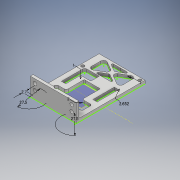
# Autodesk Inventor part: OpenMV&Ping
Saved by Autodesk Inventor 2018 (Build 220112000, 112)
## iProperties
Created: 2018-10-24
Part Number: OpenMV&Ping
Material: 一般
Document SubType Name: Modeling
Designer: shun2
Density: 1 g/cm^3
Appearance: 既定
Author: shun2
Autodesk Inventor part; units mm, degrees
ref_plane "YZ Plane" through (0, 0, 0) normal (1, 0, 0) x (0, 1, 0)
ref_plane "XZ Plane" through (0, 0, 0) normal (0, 1, 0) x (-1, 0, 0)
ref_plane "XY Plane" through (0, 0, 0) normal (0, 0, 1) x (1, 0, 0)
ref_plane "作業平面3" through (0, 0, 0) normal (0, 0, -1) x (-1, 0, 0)
sketch "スケッチ17" plane through (0, 0, 0) normal (0, 0, -1) x (-1, 0, 0)
  line L0 (19.0039, 20.5342) -> (19.0039, -23.9158)
  line L1 (19.0979, -0.4088) -> (19.0979, -12.4088)
  arc A0 (19.0661, -12.4088) -> (19.1297, -12.4088) centre (19.0979, -12.4088) ccw
  arc A1 (19.1297, -0.4088) -> (19.0661, -0.4088) centre (19.0979, -0.4088) ccw
  arc A2 (19.0979, -12.3771) -> (19.0979, -12.4406) centre (19.0979, -12.4088) ccw
  arc A3 (19.0979, -0.3771) -> (19.0979, -0.4406) centre (19.0979, -0.4088) ccw
  line L2 (1.4119, 34.5042) -> (1.4119, 35.1392)
  line L3 (-16.3681, -23.9158) -> (-16.3681, 20.5342)
  line L4 (-16.3681, 20.5342) -> (19.0039, 20.5342)
  line L5 (19.0039, -23.9158) -> (-16.3681, -23.9158)
  arc A4 (-15.9871, -20.6011) -> (-15.9871, -20.6265) centre (-15.9871, -20.6138) ccw
  arc A5 (-10.1451, -20.6265) -> (-10.1451, -20.6011) centre (-10.1451, -20.6138) ccw
  arc A6 (-13.0661, -23.5348) -> (-13.0661, -17.6928) centre (-13.0661, -20.6138) ccw
  arc A7 (-13.0661, -17.6928) -> (-13.0661, -23.5348) centre (-13.0661, -20.6138) ccw
  arc A8 (-13.0661, -22.1138) -> (-13.0661, -19.1138) centre (-13.0661, -20.6138) ccw
  arc A9 (-13.0661, -19.1138) -> (-13.0661, -22.1138) centre (-13.0661, -20.6138) ccw
  line L6 (18.8109, -20.6138) -> (18.5569, -20.6138)
  arc A10 (18.5569, -20.6011) -> (18.5569, -20.6265) centre (18.5569, -20.6138) ccw
  arc A11 (18.8109, -20.6265) -> (18.8109, -20.6011) centre (18.8109, -20.6138) ccw
  arc A12 (12.9689, -20.6011) -> (12.9689, -20.6265) centre (12.9689, -20.6138) ccw
  arc A13 (15.8899, -23.5348) -> (15.8899, -17.6928) centre (15.8899, -20.6138) ccw
  arc A14 (15.8899, -17.6928) -> (15.8899, -23.5348) centre (15.8899, -20.6138) ccw
  arc A15 (15.8899, -22.1138) -> (15.8899, -19.1138) centre (15.8899, -20.6138) ccw
  arc A16 (15.8899, -19.1138) -> (15.8899, -22.1138) centre (15.8899, -20.6138) ccw
  line L7 (18.8109, 15.8352) -> (18.8109, 17.1052)
  arc A17 (18.849, 17.1052) -> (18.7728, 17.1052) centre (18.8109, 17.1052) ccw
  arc A18 (18.7728, 15.8352) -> (18.849, 15.8352) centre (18.8109, 15.8352) ccw
  line L8 (18.8109, 17.1052) -> (18.1759, 17.7402)
  arc A19 (18.2028, 17.7671) -> (18.149, 17.7133) centre (18.1759, 17.7402) ccw
  arc A20 (18.784, 17.0783) -> (18.8378, 17.1321) centre (18.8109, 17.1052) ccw
  arc A21 (16.9059, 17.7783) -> (16.9059, 17.7021) centre (16.9059, 17.7402) ccw
  arc A22 (18.1759, 17.7021) -> (18.1759, 17.7783) centre (18.1759, 17.7402) ccw
  line L9 (16.9059, 17.7402) -> (16.2709, 17.1052)
  arc A23 (16.244, 17.1321) -> (16.2978, 17.0783) centre (16.2709, 17.1052) ccw
  arc A24 (16.9328, 17.7133) -> (16.879, 17.7671) centre (16.9059, 17.7402) ccw
  line L10 (18.1759, 12.6602) -> (18.8109, 13.2952)
  arc A25 (18.8378, 13.2683) -> (18.784, 13.3221) centre (18.8109, 13.2952) ccw
  arc A26 (18.149, 12.6871) -> (18.2028, 12.6333) centre (18.1759, 12.6602) ccw
  line L11 (18.8109, 13.2952) -> (18.8109, 14.5652)
  arc A27 (18.849, 14.5652) -> (18.7728, 14.5652) centre (18.8109, 14.5652) ccw
  arc A28 (18.7728, 13.2952) -> (18.849, 13.2952) centre (18.8109, 13.2952) ccw
  line L12 (18.8109, 14.5652) -> (18.1759, 15.2002)
  arc A29 (18.2028, 15.2271) -> (18.149, 15.1733) centre (18.1759, 15.2002) ccw
  arc A30 (18.784, 14.5383) -> (18.8378, 14.5921) centre (18.8109, 14.5652) ccw
  arc A31 (16.9059, 15.2383) -> (16.9059, 15.1621) centre (16.9059, 15.2002) ccw
  arc A32 (18.1759, 15.1621) -> (18.1759, 15.2383) centre (18.1759, 15.2002) ccw
  line L13 (16.9059, 15.2002) -> (16.2709, 14.5652)
  arc A33 (16.244, 14.5921) -> (16.2978, 14.5383) centre (16.2709, 14.5652) ccw
  arc A34 (16.9328, 15.1733) -> (16.879, 15.2271) centre (16.9059, 15.2002) ccw
  line L14 (16.2709, 14.5652) -> (16.2709, 13.2952)
  arc A35 (16.2328, 13.2952) -> (16.309, 13.2952) centre (16.2709, 13.2952) ccw
  arc A36 (16.309, 14.5652) -> (16.2328, 14.5652) centre (16.2709, 14.5652) ccw
  line L15 (16.2709, 13.2952) -> (16.9059, 12.6602)
  arc A37 (16.879, 12.6333) -> (16.9328, 12.6871) centre (16.9059, 12.6602) ccw
  arc A38 (16.2978, 13.3221) -> (16.244, 13.2683) centre (16.2709, 13.2952) ccw
  line L16 (18.8109, 15.8352) -> (18.1759, 15.2002)
  arc A39 (18.149, 15.2271) -> (18.2028, 15.1733) centre (18.1759, 15.2002) ccw
  arc A40 (18.8378, 15.8083) -> (18.784, 15.8621) centre (18.8109, 15.8352) ccw
  line L17 (16.9059, 15.2002) -> (16.2709, 15.8352)
  arc A41 (16.2978, 15.8621) -> (16.244, 15.8083) centre (16.2709, 15.8352) ccw
  arc A42 (16.879, 15.1733) -> (16.9328, 15.2271) centre (16.9059, 15.2002) ccw
  line L18 (16.2709, 17.1052) -> (16.2709, 15.8352)
  arc A43 (16.2328, 15.8352) -> (16.309, 15.8352) centre (16.2709, 15.8352) ccw
  arc A44 (16.309, 17.1052) -> (16.2328, 17.1052) centre (16.2709, 17.1052) ccw
  line L19 (18.8109, 8.2152) -> (18.8109, 9.4852)
  arc A45 (18.849, 9.4852) -> (18.7728, 9.4852) centre (18.8109, 9.4852) ccw
  arc A46 (18.7728, 8.2152) -> (18.849, 8.2152) centre (18.8109, 8.2152) ccw
  line L20 (18.8109, 9.4852) -> (18.1759, 10.1202)
  arc A47 (18.2028, 10.1471) -> (18.149, 10.0933) centre (18.1759, 10.1202) ccw
  arc A48 (18.784, 9.4583) -> (18.8378, 9.5121) centre (18.8109, 9.4852) ccw
  arc A49 (16.9059, 10.1583) -> (16.9059, 10.0821) centre (16.9059, 10.1202) ccw
  arc A50 (18.1759, 10.0821) -> (18.1759, 10.1583) centre (18.1759, 10.1202) ccw
  line L21 (16.9059, 10.1202) -> (16.2709, 9.4852)
  arc A51 (16.244, 9.5121) -> (16.2978, 9.4583) centre (16.2709, 9.4852) ccw
  arc A52 (16.9328, 10.0933) -> (16.879, 10.1471) centre (16.9059, 10.1202) ccw
  line L22 (18.1759, 10.1202) -> (18.8109, 10.7552)
  arc A53 (18.8378, 10.7283) -> (18.784, 10.7821) centre (18.8109, 10.7552) ccw
  arc A54 (18.149, 10.1471) -> (18.2028, 10.0933) centre (18.1759, 10.1202) ccw
  line L23 (18.8109, 10.7552) -> (18.8109, 12.0252)
  arc A55 (18.849, 12.0252) -> (18.7728, 12.0252) centre (18.8109, 12.0252) ccw
  arc A56 (18.7728, 10.7552) -> (18.849, 10.7552) centre (18.8109, 10.7552) ccw
  line L24 (18.8109, 12.0252) -> (18.1759, 12.6602)
  arc A57 (18.2028, 12.6871) -> (18.149, 12.6333) centre (18.1759, 12.6602) ccw
  arc A58 (18.784, 11.9983) -> (18.8378, 12.0521) centre (18.8109, 12.0252) ccw
  arc A59 (16.9059, 12.6983) -> (16.9059, 12.6221) centre (16.9059, 12.6602) ccw
  arc A60 (18.1759, 12.6221) -> (18.1759, 12.6983) centre (18.1759, 12.6602) ccw
  line L25 (16.9059, 12.6602) -> (16.2709, 12.0252)
  arc A61 (16.244, 12.0521) -> (16.2978, 11.9983) centre (16.2709, 12.0252) ccw
  arc A62 (16.9328, 12.6333) -> (16.879, 12.6871) centre (16.9059, 12.6602) ccw
  line L26 (16.2709, 12.0252) -> (16.2709, 10.7552)
  arc A63 (16.2328, 10.7552) -> (16.309, 10.7552) centre (16.2709, 10.7552) ccw
  arc A64 (16.309, 12.0252) -> (16.2328, 12.0252) centre (16.2709, 12.0252) ccw
  line L27 (16.2709, 10.7552) -> (16.9059, 10.1202)
  arc A65 (16.879, 10.0933) -> (16.9328, 10.1471) centre (16.9059, 10.1202) ccw
  arc A66 (16.2978, 10.7821) -> (16.244, 10.7283) centre (16.2709, 10.7552) ccw
  line L28 (18.1759, 5.0402) -> (18.8109, 5.6752)
  arc A67 (18.8378, 5.6483) -> (18.784, 5.7021) centre (18.8109, 5.6752) ccw
  arc A68 (18.149, 5.0671) -> (18.2028, 5.0133) centre (18.1759, 5.0402) ccw
  line L29 (18.8109, 5.6752) -> (18.8109, 6.9452)
  arc A69 (18.849, 6.9452) -> (18.7728, 6.9452) centre (18.8109, 6.9452) ccw
  arc A70 (18.7728, 5.6752) -> (18.849, 5.6752) centre (18.8109, 5.6752) ccw
  line L30 (18.8109, 6.9452) -> (18.1759, 7.5802)
  arc A71 (18.2028, 7.6071) -> (18.149, 7.5533) centre (18.1759, 7.5802) ccw
  arc A72 (18.784, 6.9183) -> (18.8378, 6.9721) centre (18.8109, 6.9452) ccw
  arc A73 (16.9059, 7.6183) -> (16.9059, 7.5421) centre (16.9059, 7.5802) ccw
  arc A74 (18.1759, 7.5421) -> (18.1759, 7.6183) centre (18.1759, 7.5802) ccw
  line L31 (16.9059, 7.5802) -> (16.2709, 6.9452)
  arc A75 (16.244, 6.9721) -> (16.2978, 6.9183) centre (16.2709, 6.9452) ccw
  arc A76 (16.9328, 7.5533) -> (16.879, 7.6071) centre (16.9059, 7.5802) ccw
  line L32 (16.2709, 6.9452) -> (16.2709, 5.6752)
  arc A77 (16.2328, 5.6752) -> (16.309, 5.6752) centre (16.2709, 5.6752) ccw
  arc A78 (16.309, 6.9452) -> (16.2328, 6.9452) centre (16.2709, 6.9452) ccw
  line L33 (16.2709, 5.6752) -> (16.9059, 5.0402)
  arc A79 (16.879, 5.0133) -> (16.9328, 5.0671) centre (16.9059, 5.0402) ccw
  arc A80 (16.2978, 5.7021) -> (16.244, 5.6483) centre (16.2709, 5.6752) ccw
  line L34 (18.8109, 8.2152) -> (18.1759, 7.5802)
  arc A81 (18.149, 7.6071) -> (18.2028, 7.5533) centre (18.1759, 7.5802) ccw
  arc A82 (18.8378, 8.1883) -> (18.784, 8.2421) centre (18.8109, 8.2152) ccw
  line L35 (16.9059, 7.5802) -> (16.2709, 8.2152)
  arc A83 (16.2978, 8.2421) -> (16.244, 8.1883) centre (16.2709, 8.2152) ccw
  arc A84 (16.879, 7.5533) -> (16.9328, 7.6071) centre (16.9059, 7.5802) ccw
  line L36 (16.2709, 9.4852) -> (16.2709, 8.2152)
  arc A85 (16.2328, 8.2152) -> (16.309, 8.2152) centre (16.2709, 8.2152) ccw
  arc A86 (16.309, 9.4852) -> (16.2328, 9.4852) centre (16.2709, 9.4852) ccw
  line L37 (18.8109, 0.5952) -> (18.8109, 1.8652)
  arc A87 (18.849, 1.8652) -> (18.7728, 1.8652) centre (18.8109, 1.8652) ccw
  arc A88 (18.7728, 0.5952) -> (18.849, 0.5952) centre (18.8109, 0.5952) ccw
  line L38 (18.8109, 1.8652) -> (18.1759, 2.5002)
  arc A89 (18.2028, 2.5271) -> (18.149, 2.4733) centre (18.1759, 2.5002) ccw
  arc A90 (18.784, 1.8383) -> (18.8378, 1.8921) centre (18.8109, 1.8652) ccw
  arc A91 (16.9059, 2.5383) -> (16.9059, 2.4621) centre (16.9059, 2.5002) ccw
  arc A92 (18.1759, 2.4621) -> (18.1759, 2.5383) centre (18.1759, 2.5002) ccw
  line L39 (16.9059, 2.5002) -> (16.2709, 1.8652)
  arc A93 (16.244, 1.8921) -> (16.2978, 1.8383) centre (16.2709, 1.8652) ccw
  arc A94 (16.9328, 2.4733) -> (16.879, 2.5271) centre (16.9059, 2.5002) ccw
  line L40 (18.1759, 2.5002) -> (18.8109, 3.1352)
  arc A95 (18.8378, 3.1083) -> (18.784, 3.1621) centre (18.8109, 3.1352) ccw
  arc A96 (18.149, 2.5271) -> (18.2028, 2.4733) centre (18.1759, 2.5002) ccw
  line L41 (18.8109, 3.1352) -> (18.8109, 4.4052)
  arc A97 (18.849, 4.4052) -> (18.7728, 4.4052) centre (18.8109, 4.4052) ccw
  arc A98 (18.7728, 3.1352) -> (18.849, 3.1352) centre (18.8109, 3.1352) ccw
  line L42 (18.8109, 4.4052) -> (18.1759, 5.0402)
  arc A99 (18.2028, 5.0671) -> (18.149, 5.0133) centre (18.1759, 5.0402) ccw
  arc A100 (18.784, 4.3783) -> (18.8378, 4.4321) centre (18.8109, 4.4052) ccw
  arc A101 (16.9059, 5.0783) -> (16.9059, 5.0021) centre (16.9059, 5.0402) ccw
  arc A102 (18.1759, 5.0021) -> (18.1759, 5.0783) centre (18.1759, 5.0402) ccw
  line L43 (16.9059, 5.0402) -> (16.2709, 4.4052)
  arc A103 (16.244, 4.4321) -> (16.2978, 4.3783) centre (16.2709, 4.4052) ccw
  arc A104 (16.9328, 5.0133) -> (16.879, 5.0671) centre (16.9059, 5.0402) ccw
  line L44 (16.2709, 4.4052) -> (16.2709, 3.1352)
  arc A105 (16.2328, 3.1352) -> (16.309, 3.1352) centre (16.2709, 3.1352) ccw
  arc A106 (16.309, 4.4052) -> (16.2328, 4.4052) centre (16.2709, 4.4052) ccw
  line L45 (16.2709, 3.1352) -> (16.9059, 2.5002)
  arc A107 (16.879, 2.4733) -> (16.9328, 2.5271) centre (16.9059, 2.5002) ccw
  arc A108 (16.2978, 3.1621) -> (16.244, 3.1083) centre (16.2709, 3.1352) ccw
  line L46 (18.1759, -0.0398) -> (16.9059, -0.0398)
  arc A109 (16.9059, -0.0017) -> (16.9059, -0.0779) centre (16.9059, -0.0398) ccw
  arc A110 (18.1759, -0.0779) -> (18.1759, -0.0017) centre (18.1759, -0.0398) ccw
  line L47 (18.8109, 0.5952) -> (18.1759, -0.0398)
  arc A111 (18.149, -0.0129) -> (18.2028, -0.0667) centre (18.1759, -0.0398) ccw
  arc A112 (18.8378, 0.5683) -> (18.784, 0.6221) centre (18.8109, 0.5952) ccw
  line L48 (16.9059, -0.0398) -> (16.2709, 0.5952)
  arc A113 (16.2978, 0.6221) -> (16.244, 0.5683) centre (16.2709, 0.5952) ccw
  arc A114 (16.879, -0.0667) -> (16.9328, -0.0129) centre (16.9059, -0.0398) ccw
  line L49 (16.2709, 1.8652) -> (16.2709, 0.5952)
  arc A115 (16.2328, 0.5952) -> (16.309, 0.5952) centre (16.2709, 0.5952) ccw
  arc A116 (16.309, 1.8652) -> (16.2328, 1.8652) centre (16.2709, 1.8652) ccw
  line L50 (18.8109, 18.3752) -> (18.8109, 19.6452)
  arc A117 (18.849, 19.6452) -> (18.7728, 19.6452) centre (18.8109, 19.6452) ccw
  arc A118 (18.7728, 18.3752) -> (18.849, 18.3752) centre (18.8109, 18.3752) ccw
  line L51 (18.8109, 19.6452) -> (18.1759, 20.2802)
  arc A119 (18.2028, 20.3071) -> (18.149, 20.2533) centre (18.1759, 20.2802) ccw
  arc A120 (18.784, 19.6183) -> (18.8378, 19.6721) centre (18.8109, 19.6452) ccw
  line L52 (18.1759, 20.2802) -> (16.9059, 20.2802)
  arc A121 (16.9059, 20.3183) -> (16.9059, 20.2421) centre (16.9059, 20.2802) ccw
  arc A122 (18.1759, 20.2421) -> (18.1759, 20.3183) centre (18.1759, 20.2802) ccw
  line L53 (16.9059, 20.2802) -> (16.2709, 19.6452)
  arc A123 (16.244, 19.6721) -> (16.2978, 19.6183) centre (16.2709, 19.6452) ccw
  arc A124 (16.9328, 20.2533) -> (16.879, 20.3071) centre (16.9059, 20.2802) ccw
  line L54 (18.8109, 18.3752) -> (18.1759, 17.7402)
  arc A125 (18.149, 17.7671) -> (18.2028, 17.7133) centre (18.1759, 17.7402) ccw
  arc A126 (18.8378, 18.3483) -> (18.784, 18.4021) centre (18.8109, 18.3752) ccw
  line L55 (16.9059, 17.7402) -> (16.2709, 18.3752)
  arc A127 (16.2978, 18.4021) -> (16.244, 18.3483) centre (16.2709, 18.3752) ccw
  arc A128 (16.879, 17.7133) -> (16.9328, 17.7671) centre (16.9059, 17.7402) ccw
  line L56 (16.2709, 19.6452) -> (16.2709, 18.3752)
  arc A129 (16.2328, 18.3752) -> (16.309, 18.3752) centre (16.2709, 18.3752) ccw
  arc A130 (16.309, 19.6452) -> (16.2328, 19.6452) centre (16.2709, 19.6452) ccw
  line L57 (-13.4471, 15.8352) -> (-13.4471, 17.1052)
  arc A131 (-13.409, 17.1052) -> (-13.4852, 17.1052) centre (-13.4471, 17.1052) ccw
  arc A132 (-13.4852, 15.8352) -> (-13.409, 15.8352) centre (-13.4471, 15.8352) ccw
  line L58 (-13.4471, 17.1052) -> (-14.0821, 17.7402)
  arc A133 (-14.0552, 17.7671) -> (-14.109, 17.7133) centre (-14.0821, 17.7402) ccw
  arc A134 (-13.474, 17.0783) -> (-13.4202, 17.1321) centre (-13.4471, 17.1052) ccw
  arc A135 (-15.3521, 17.7783) -> (-15.3521, 17.7021) centre (-15.3521, 17.7402) ccw
  arc A136 (-14.0821, 17.7021) -> (-14.0821, 17.7783) centre (-14.0821, 17.7402) ccw
  line L59 (-15.3521, 17.7402) -> (-15.9871, 17.1052)
  arc A137 (-16.014, 17.1321) -> (-15.9602, 17.0783) centre (-15.9871, 17.1052) ccw
  arc A138 (-15.3252, 17.7133) -> (-15.379, 17.7671) centre (-15.3521, 17.7402) ccw
  line L60 (-14.0821, 12.6602) -> (-13.4471, 13.2952)
  arc A139 (-13.4202, 13.2683) -> (-13.474, 13.3221) centre (-13.4471, 13.2952) ccw
  arc A140 (-14.109, 12.6871) -> (-14.0552, 12.6333) centre (-14.0821, 12.6602) ccw
  line L61 (-13.4471, 13.2952) -> (-13.4471, 14.5652)
  arc A141 (-13.409, 14.5652) -> (-13.4852, 14.5652) centre (-13.4471, 14.5652) ccw
  arc A142 (-13.4852, 13.2952) -> (-13.409, 13.2952) centre (-13.4471, 13.2952) ccw
  line L62 (-13.4471, 14.5652) -> (-14.0821, 15.2002)
  arc A143 (-14.0552, 15.2271) -> (-14.109, 15.1733) centre (-14.0821, 15.2002) ccw
  arc A144 (-13.474, 14.5383) -> (-13.4202, 14.5921) centre (-13.4471, 14.5652) ccw
  arc A145 (-15.3521, 15.2383) -> (-15.3521, 15.1621) centre (-15.3521, 15.2002) ccw
  arc A146 (-14.0821, 15.1621) -> (-14.0821, 15.2383) centre (-14.0821, 15.2002) ccw
  line L63 (-15.3521, 15.2002) -> (-15.9871, 14.5652)
  arc A147 (-16.014, 14.5921) -> (-15.9602, 14.5383) centre (-15.9871, 14.5652) ccw
  arc A148 (-15.3252, 15.1733) -> (-15.379, 15.2271) centre (-15.3521, 15.2002) ccw
  line L64 (-15.9871, 14.5652) -> (-15.9871, 13.2952)
  arc A149 (-16.0252, 13.2952) -> (-15.949, 13.2952) centre (-15.9871, 13.2952) ccw
  arc A150 (-15.949, 14.5652) -> (-16.0252, 14.5652) centre (-15.9871, 14.5652) ccw
  line L65 (-15.9871, 13.2952) -> (-15.3521, 12.6602)
  arc A151 (-15.379, 12.6333) -> (-15.3252, 12.6871) centre (-15.3521, 12.6602) ccw
  arc A152 (-15.9602, 13.3221) -> (-16.014, 13.2683) centre (-15.9871, 13.2952) ccw
  line L66 (-13.4471, 15.8352) -> (-14.0821, 15.2002)
  arc A153 (-14.109, 15.2271) -> (-14.0552, 15.1733) centre (-14.0821, 15.2002) ccw
  arc A154 (-13.4202, 15.8083) -> (-13.474, 15.8621) centre (-13.4471, 15.8352) ccw
  line L67 (-15.3521, 15.2002) -> (-15.9871, 15.8352)
  arc A155 (-15.9602, 15.8621) -> (-16.014, 15.8083) centre (-15.9871, 15.8352) ccw
  arc A156 (-15.379, 15.1733) -> (-15.3252, 15.2271) centre (-15.3521, 15.2002) ccw
  line L68 (-15.9871, 17.1052) -> (-15.9871, 15.8352)
  arc A157 (-16.0252, 15.8352) -> (-15.949, 15.8352) centre (-15.9871, 15.8352) ccw
  arc A158 (-15.949, 17.1052) -> (-16.0252, 17.1052) centre (-15.9871, 17.1052) ccw
  line L69 (-13.4471, 8.2152) -> (-13.4471, 9.4852)
  arc A159 (-13.409, 9.4852) -> (-13.4852, 9.4852) centre (-13.4471, 9.4852) ccw
  arc A160 (-13.4852, 8.2152) -> (-13.409, 8.2152) centre (-13.4471, 8.2152) ccw
  line L70 (-13.4471, 9.4852) -> (-14.0821, 10.1202)
  arc A161 (-14.0552, 10.1471) -> (-14.109, 10.0933) centre (-14.0821, 10.1202) ccw
  arc A162 (-13.474, 9.4583) -> (-13.4202, 9.5121) centre (-13.4471, 9.4852) ccw
  arc A163 (-15.3521, 10.1583) -> (-15.3521, 10.0821) centre (-15.3521, 10.1202) ccw
  arc A164 (-14.0821, 10.0821) -> (-14.0821, 10.1583) centre (-14.0821, 10.1202) ccw
  line L71 (-15.3521, 10.1202) -> (-15.9871, 9.4852)
  arc A165 (-16.014, 9.5121) -> (-15.9602, 9.4583) centre (-15.9871, 9.4852) ccw
  arc A166 (-15.3252, 10.0933) -> (-15.379, 10.1471) centre (-15.3521, 10.1202) ccw
  line L72 (-14.0821, 10.1202) -> (-13.4471, 10.7552)
  arc A167 (-13.4202, 10.7283) -> (-13.474, 10.7821) centre (-13.4471, 10.7552) ccw
  arc A168 (-14.109, 10.1471) -> (-14.0552, 10.0933) centre (-14.0821, 10.1202) ccw
  line L73 (-13.4471, 10.7552) -> (-13.4471, 12.0252)
  arc A169 (-13.409, 12.0252) -> (-13.4852, 12.0252) centre (-13.4471, 12.0252) ccw
  arc A170 (-13.4852, 10.7552) -> (-13.409, 10.7552) centre (-13.4471, 10.7552) ccw
  line L74 (-13.4471, 12.0252) -> (-14.0821, 12.6602)
  arc A171 (-14.0552, 12.6871) -> (-14.109, 12.6333) centre (-14.0821, 12.6602) ccw
  arc A172 (-13.474, 11.9983) -> (-13.4202, 12.0521) centre (-13.4471, 12.0252) ccw
  arc A173 (-15.3521, 12.6983) -> (-15.3521, 12.6221) centre (-15.3521, 12.6602) ccw
  arc A174 (-14.0821, 12.6221) -> (-14.0821, 12.6983) centre (-14.0821, 12.6602) ccw
  line L75 (-15.3521, 12.6602) -> (-15.9871, 12.0252)
  arc A175 (-16.014, 12.0521) -> (-15.9602, 11.9983) centre (-15.9871, 12.0252) ccw
  arc A176 (-15.3252, 12.6333) -> (-15.379, 12.6871) centre (-15.3521, 12.6602) ccw
  line L76 (-15.9871, 12.0252) -> (-15.9871, 10.7552)
  arc A177 (-16.0252, 10.7552) -> (-15.949, 10.7552) centre (-15.9871, 10.7552) ccw
  arc A178 (-15.949, 12.0252) -> (-16.0252, 12.0252) centre (-15.9871, 12.0252) ccw
  line L77 (-15.9871, 10.7552) -> (-15.3521, 10.1202)
  arc A179 (-15.379, 10.0933) -> (-15.3252, 10.1471) centre (-15.3521, 10.1202) ccw
  arc A180 (-15.9602, 10.7821) -> (-16.014, 10.7283) centre (-15.9871, 10.7552) ccw
  line L78 (-14.0821, 5.0402) -> (-13.4471, 5.6752)
  arc A181 (-13.4202, 5.6483) -> (-13.474, 5.7021) centre (-13.4471, 5.6752) ccw
  arc A182 (-14.109, 5.0671) -> (-14.0552, 5.0133) centre (-14.0821, 5.0402) ccw
  line L79 (-13.4471, 5.6752) -> (-13.4471, 6.9452)
  arc A183 (-13.409, 6.9452) -> (-13.4852, 6.9452) centre (-13.4471, 6.9452) ccw
  arc A184 (-13.4852, 5.6752) -> (-13.409, 5.6752) centre (-13.4471, 5.6752) ccw
  line L80 (-13.4471, 6.9452) -> (-14.0821, 7.5802)
  arc A185 (-14.0552, 7.6071) -> (-14.109, 7.5533) centre (-14.0821, 7.5802) ccw
  arc A186 (-13.474, 6.9183) -> (-13.4202, 6.9721) centre (-13.4471, 6.9452) ccw
  arc A187 (-15.3521, 7.6183) -> (-15.3521, 7.5421) centre (-15.3521, 7.5802) ccw
  arc A188 (-14.0821, 7.5421) -> (-14.0821, 7.6183) centre (-14.0821, 7.5802) ccw
  line L81 (-15.3521, 7.5802) -> (-15.9871, 6.9452)
  arc A189 (-16.014, 6.9721) -> (-15.9602, 6.9183) centre (-15.9871, 6.9452) ccw
  arc A190 (-15.3252, 7.5533) -> (-15.379, 7.6071) centre (-15.3521, 7.5802) ccw
  line L82 (-15.9871, 6.9452) -> (-15.9871, 5.6752)
  arc A191 (-16.0252, 5.6752) -> (-15.949, 5.6752) centre (-15.9871, 5.6752) ccw
  arc A192 (-15.949, 6.9452) -> (-16.0252, 6.9452) centre (-15.9871, 6.9452) ccw
  line L83 (-15.9871, 5.6752) -> (-15.3521, 5.0402)
  arc A193 (-15.379, 5.0133) -> (-15.3252, 5.0671) centre (-15.3521, 5.0402) ccw
  arc A194 (-15.9602, 5.7021) -> (-16.014, 5.6483) centre (-15.9871, 5.6752) ccw
  line L84 (-13.4471, 8.2152) -> (-14.0821, 7.5802)
  arc A195 (-14.109, 7.6071) -> (-14.0552, 7.5533) centre (-14.0821, 7.5802) ccw
  arc A196 (-13.4202, 8.1883) -> (-13.474, 8.2421) centre (-13.4471, 8.2152) ccw
  line L85 (-15.3521, 7.5802) -> (-15.9871, 8.2152)
  arc A197 (-15.9602, 8.2421) -> (-16.014, 8.1883) centre (-15.9871, 8.2152) ccw
  arc A198 (-15.379, 7.5533) -> (-15.3252, 7.6071) centre (-15.3521, 7.5802) ccw
  line L86 (-15.9871, 9.4852) -> (-15.9871, 8.2152)
  arc A199 (-16.0252, 8.2152) -> (-15.949, 8.2152) centre (-15.9871, 8.2152) ccw
  arc A200 (-15.949, 9.4852) -> (-16.0252, 9.4852) centre (-15.9871, 9.4852) ccw
  line L87 (-13.4471, 0.5952) -> (-13.4471, 1.8652)
  arc A201 (-13.409, 1.8652) -> (-13.4852, 1.8652) centre (-13.4471, 1.8652) ccw
  arc A202 (-13.4852, 0.5952) -> (-13.409, 0.5952) centre (-13.4471, 0.5952) ccw
  line L88 (-13.4471, 1.8652) -> (-14.0821, 2.5002)
  arc A203 (-14.0552, 2.5271) -> (-14.109, 2.4733) centre (-14.0821, 2.5002) ccw
  arc A204 (-13.474, 1.8383) -> (-13.4202, 1.8921) centre (-13.4471, 1.8652) ccw
  arc A205 (-15.3521, 2.5383) -> (-15.3521, 2.4621) centre (-15.3521, 2.5002) ccw
  arc A206 (-14.0821, 2.4621) -> (-14.0821, 2.5383) centre (-14.0821, 2.5002) ccw
  line L89 (-15.3521, 2.5002) -> (-15.9871, 1.8652)
  arc A207 (-16.014, 1.8921) -> (-15.9602, 1.8383) centre (-15.9871, 1.8652) ccw
  arc A208 (-15.3252, 2.4733) -> (-15.379, 2.5271) centre (-15.3521, 2.5002) ccw
  line L90 (-14.0821, 2.5002) -> (-13.4471, 3.1352)
  arc A209 (-13.4202, 3.1083) -> (-13.474, 3.1621) centre (-13.4471, 3.1352) ccw
  arc A210 (-14.109, 2.5271) -> (-14.0552, 2.4733) centre (-14.0821, 2.5002) ccw
  line L91 (-13.4471, 3.1352) -> (-13.4471, 4.4052)
  arc A211 (-13.409, 4.4052) -> (-13.4852, 4.4052) centre (-13.4471, 4.4052) ccw
  arc A212 (-13.4852, 3.1352) -> (-13.409, 3.1352) centre (-13.4471, 3.1352) ccw
  line L92 (-13.4471, 4.4052) -> (-14.0821, 5.0402)
  arc A213 (-14.0552, 5.0671) -> (-14.109, 5.0133) centre (-14.0821, 5.0402) ccw
  arc A214 (-13.474, 4.3783) -> (-13.4202, 4.4321) centre (-13.4471, 4.4052) ccw
  arc A215 (-15.3521, 5.0783) -> (-15.3521, 5.0021) centre (-15.3521, 5.0402) ccw
  arc A216 (-14.0821, 5.0021) -> (-14.0821, 5.0783) centre (-14.0821, 5.0402) ccw
  line L93 (-15.3521, 5.0402) -> (-15.9871, 4.4052)
  arc A217 (-16.014, 4.4321) -> (-15.9602, 4.3783) centre (-15.9871, 4.4052) ccw
  arc A218 (-15.3252, 5.0133) -> (-15.379, 5.0671) centre (-15.3521, 5.0402) ccw
  line L94 (-15.9871, 4.4052) -> (-15.9871, 3.1352)
  arc A219 (-16.0252, 3.1352) -> (-15.949, 3.1352) centre (-15.9871, 3.1352) ccw
  arc A220 (-15.949, 4.4052) -> (-16.0252, 4.4052) centre (-15.9871, 4.4052) ccw
  line L95 (-15.9871, 3.1352) -> (-15.3521, 2.5002)
  arc A221 (-15.379, 2.4733) -> (-15.3252, 2.5271) centre (-15.3521, 2.5002) ccw
  arc A222 (-15.9602, 3.1621) -> (-16.014, 3.1083) centre (-15.9871, 3.1352) ccw
  line L96 (-14.0821, -0.0398) -> (-15.3521, -0.0398)
  arc A223 (-15.3521, -0.0017) -> (-15.3521, -0.0779) centre (-15.3521, -0.0398) ccw
  arc A224 (-14.0821, -0.0779) -> (-14.0821, -0.0017) centre (-14.0821, -0.0398) ccw
  line L97 (-13.4471, 0.5952) -> (-14.0821, -0.0398)
  arc A225 (-14.109, -0.0129) -> (-14.0552, -0.0667) centre (-14.0821, -0.0398) ccw
  arc A226 (-13.4202, 0.5683) -> (-13.474, 0.6221) centre (-13.4471, 0.5952) ccw
  line L98 (-15.3521, -0.0398) -> (-15.9871, 0.5952)
  arc A227 (-15.9602, 0.6221) -> (-16.014, 0.5683) centre (-15.9871, 0.5952) ccw
  arc A228 (-15.379, -0.0667) -> (-15.3252, -0.0129) centre (-15.3521, -0.0398) ccw
  line L99 (-15.9871, 1.8652) -> (-15.9871, 0.5952)
  arc A229 (-16.0252, 0.5952) -> (-15.949, 0.5952) centre (-15.9871, 0.5952) ccw
  arc A230 (-15.949, 1.8652) -> (-16.0252, 1.8652) centre (-15.9871, 1.8652) ccw
  line L100 (-13.4471, 18.3752) -> (-13.4471, 19.6452)
  arc A231 (-13.409, 19.6452) -> (-13.4852, 19.6452) centre (-13.4471, 19.6452) ccw
  arc A232 (-13.4852, 18.3752) -> (-13.409, 18.3752) centre (-13.4471, 18.3752) ccw
  line L101 (-13.4471, 19.6452) -> (-14.0821, 20.2802)
  arc A233 (-14.0552, 20.3071) -> (-14.109, 20.2533) centre (-14.0821, 20.2802) ccw
  arc A234 (-13.474, 19.6183) -> (-13.4202, 19.6721) centre (-13.4471, 19.6452) ccw
  line L102 (-14.0821, 20.2802) -> (-15.3521, 20.2802)
  arc A235 (-15.3521, 20.3183) -> (-15.3521, 20.2421) centre (-15.3521, 20.2802) ccw
  arc A236 (-14.0821, 20.2421) -> (-14.0821, 20.3183) centre (-14.0821, 20.2802) ccw
  line L103 (-15.3521, 20.2802) -> (-15.9871, 19.6452)
  arc A237 (-16.014, 19.6721) -> (-15.9602, 19.6183) centre (-15.9871, 19.6452) ccw
  arc A238 (-15.3252, 20.2533) -> (-15.379, 20.3071) centre (-15.3521, 20.2802) ccw
  line L104 (-13.4471, 18.3752) -> (-14.0821, 17.7402)
  arc A239 (-14.109, 17.7671) -> (-14.0552, 17.7133) centre (-14.0821, 17.7402) ccw
  arc A240 (-13.4202, 18.3483) -> (-13.474, 18.4021) centre (-13.4471, 18.3752) ccw
  line L105 (-15.3521, 17.7402) -> (-15.9871, 18.3752)
  arc A241 (-15.9602, 18.4021) -> (-16.014, 18.3483) centre (-15.9871, 18.3752) ccw
  arc A242 (-15.379, 17.7133) -> (-15.3252, 17.7671) centre (-15.3521, 17.7402) ccw
  line L106 (-15.9871, 19.6452) -> (-15.9871, 18.3752)
  arc A243 (-16.0252, 18.3752) -> (-15.949, 18.3752) centre (-15.9871, 18.3752) ccw
  arc A244 (-15.949, 19.6452) -> (-16.0252, 19.6452) centre (-15.9871, 19.6452) ccw
  line L107 (-15.1281, -10.8648) -> (-15.4281, -10.8648)
  arc A245 (-15.4281, -10.814) -> (-15.4281, -10.9156) centre (-15.4281, -10.8648) ccw
  arc A246 (-15.1281, -10.9156) -> (-15.1281, -10.814) centre (-15.1281, -10.8648) ccw
  line L108 (-15.4281, -10.8648) -> (-15.4281, -8.2648)
  arc A247 (-15.3773, -8.2648) -> (-15.4789, -8.2648) centre (-15.4281, -8.2648) ccw
  arc A248 (-15.4789, -10.8648) -> (-15.3773, -10.8648) centre (-15.4281, -10.8648) ccw
  line L109 (-15.4281, -8.2648) -> (-15.1281, -8.2648)
  arc A249 (-15.1281, -8.3156) -> (-15.1281, -8.214) centre (-15.1281, -8.2648) ccw
  arc A250 (-15.4281, -8.214) -> (-15.4281, -8.3156) centre (-15.4281, -8.2648) ccw
  line L110 (-12.5281, -10.8648) -> (-12.2281, -10.8648)
  arc A251 (-12.2281, -10.9156) -> (-12.2281, -10.814) centre (-12.2281, -10.8648) ccw
  arc A252 (-12.5281, -10.814) -> (-12.5281, -10.9156) centre (-12.5281, -10.8648) ccw
  line L111 (-12.2281, -10.8648) -> (-12.2281, -8.2648)
  arc A253 (-12.1773, -8.2648) -> (-12.2789, -8.2648) centre (-12.2281, -8.2648) ccw
  arc A254 (-12.2789, -10.8648) -> (-12.1773, -10.8648) centre (-12.2281, -10.8648) ccw
  line L112 (-12.2281, -8.2648) -> (-12.5281, -8.2648)
  arc A255 (-12.5281, -8.214) -> (-12.5281, -8.3156) centre (-12.5281, -8.2648) ccw
  arc A256 (-12.2281, -8.3156) -> (-12.2281, -8.214) centre (-12.2281, -8.2648) ccw
  line L113 (-6.5881, -7.5338) -> (-6.5881, -13.5568)
  arc A257 (-6.6198, -13.5568) -> (-6.5563, -13.5568) centre (-6.5881, -13.5568) ccw
  arc A258 (-6.5563, -7.5338) -> (-6.6198, -7.5338) centre (-6.5881, -7.5338) ccw
  line L114 (-6.5881, -13.5568) -> (-6.5881, -17.5108)
  arc A259 (-6.6198, -17.5108) -> (-6.5563, -17.5108) centre (-6.5881, -17.5108) ccw
  arc A260 (-6.5563, -13.5568) -> (-6.6198, -13.5568) centre (-6.5881, -13.5568) ccw
  line L115 (-6.5881, -17.5108) -> (-6.5881, -23.5338)
  arc A261 (-6.6198, -23.5338) -> (-6.5563, -23.5338) centre (-6.5881, -23.5338) ccw
  arc A262 (-6.5563, -17.5108) -> (-6.6198, -17.5108) centre (-6.5881, -17.5108) ccw
  line L116 (-6.5881, -23.5338) -> (9.4119, -23.5338)
  arc A263 (9.4119, -23.5656) -> (9.4119, -23.5021) centre (9.4119, -23.5338) ccw
  arc A264 (-6.5881, -23.5021) -> (-6.5881, -23.5656) centre (-6.5881, -23.5338) ccw
  line L117 (9.4119, -23.5338) -> (9.4119, -17.5108)
  arc A265 (9.4436, -17.5108) -> (9.3802, -17.5108) centre (9.4119, -17.5108) ccw
  arc A266 (9.3802, -23.5338) -> (9.4436, -23.5338) centre (9.4119, -23.5338) ccw
  line L118 (9.4119, -17.5108) -> (9.4119, -13.5568)
  arc A267 (9.4436, -13.5568) -> (9.3802, -13.5568) centre (9.4119, -13.5568) ccw
  arc A268 (9.3802, -17.5108) -> (9.4436, -17.5108) centre (9.4119, -17.5108) ccw
  line L119 (9.4119, -13.5568) -> (9.4119, -7.5338)
  arc A269 (9.4436, -7.5338) -> (9.3802, -7.5338) centre (9.4119, -7.5338) ccw
  arc A270 (9.3802, -13.5568) -> (9.4436, -13.5568) centre (9.4119, -13.5568) ccw
  line L120 (9.4119, -7.5338) -> (-6.5881, -7.5338)
  arc A271 (-6.5881, -7.5021) -> (-6.5881, -7.5656) centre (-6.5881, -7.5338) ccw
  arc A272 (9.4119, -7.5656) -> (9.4119, -7.5021) centre (9.4119, -7.5338) ccw
  arc A273 (-6.5881, -13.5568) -> (-6.5881, -17.5108) centre (-8.5651, -15.5338) ccw
  arc A274 (-6.5656, -17.5333) -> (-6.6106, -17.4883) centre (-6.5881, -17.5108) ccw
  arc A275 (-6.6106, -13.5793) -> (-6.5656, -13.5343) centre (-6.5881, -13.5568) ccw
  arc A276 (9.4119, -17.5108) -> (9.4119, -13.5568) centre (11.3888, -15.5338) ccw
  arc A277 (9.3894, -13.5343) -> (9.4344, -13.5793) centre (9.4119, -13.5568) ccw
  arc A278 (9.4344, -17.4883) -> (9.3894, -17.5333) centre (9.4119, -17.5108) ccw
  arc A279 (19.0661, -12.4088) -> (19.1297, -12.4088) centre (19.0979, -12.4088) ccw
  arc A280 (19.1297, -0.4088) -> (19.0661, -0.4088) centre (19.0979, -0.4088) ccw
  line L121 (19.0979, -12.4088) -> (13.4979, -12.4088)
  arc A281 (13.4979, -12.3771) -> (13.4979, -12.4406) centre (13.4979, -12.4088) ccw
  arc A282 (19.0979, -12.4406) -> (19.0979, -12.3771) centre (19.0979, -12.4088) ccw
  line L122 (13.4979, -12.4088) -> (13.4979, -0.4088)
  arc A283 (13.4662, -12.4088) -> (13.5296, -12.4088) centre (13.4979, -12.4088) ccw
  line L123 (13.4979, -0.4088) -> (19.0979, -0.4088)
  arc A284 (19.0979, -0.4406) -> (19.0979, -0.3771) centre (19.0979, -0.4088) ccw
  line L124 (5.7219, 20.5317) -> (14.8819, 20.5317)
  arc A285 (14.8819, 20.4999) -> (14.8819, 20.5635) centre (14.8819, 20.5317) ccw
  arc A286 (5.7219, 20.5635) -> (5.7219, 20.4999) centre (5.7219, 20.5317) ccw
  line L125 (5.7219, 20.5317) -> (5.7219, 15.3767)
  arc A287 (5.6902, 15.3767) -> (5.7536, 15.3767) centre (5.7219, 15.3767) ccw
  arc A288 (5.7536, 20.5317) -> (5.6902, 20.5317) centre (5.7219, 20.5317) ccw
  line L126 (5.7219, 15.3767) -> (14.8819, 15.3767)
  arc A289 (14.8819, 15.3449) -> (14.8819, 15.4084) centre (14.8819, 15.3767) ccw
  arc A290 (5.7219, 15.4084) -> (5.7219, 15.3449) centre (5.7219, 15.3767) ccw
  line L127 (14.8819, 15.3767) -> (14.8819, 20.5317)
  arc A291 (14.9136, 20.5317) -> (14.8502, 20.5317) centre (14.8819, 20.5317) ccw
  arc A292 (14.8502, 15.3767) -> (14.9136, 15.3767) centre (14.8819, 15.3767) ccw
  arc A293 (-8.4941, -22.7688) -> (-8.4941, -22.2688) centre (-8.4941, -22.5188) ccw
  arc A294 (-8.4941, -22.2688) -> (-8.4941, -22.7688) centre (-8.4941, -22.5188) ccw
  arc A295 (-8.4941, -22.7688) -> (-8.4941, -22.2688) centre (-8.4941, -22.5188) ccw
  arc A296 (-8.4941, -22.2688) -> (-8.4941, -22.7688) centre (-8.4941, -22.5188) ccw
  arc A297 (-14.3996, -20.6138) -> (-11.7326, -20.6138) centre (-13.0661, -20.6138) ccw
  arc A298 (-11.7326, -20.6138) -> (-14.3996, -20.6138) centre (-13.0661, -20.6138) ccw
  arc A299 (-14.0201, -20.6138) -> (-12.1121, -20.6138) centre (-13.0661, -20.6138) ccw
  arc A300 (-12.1121, -20.6138) -> (-14.0201, -20.6138) centre (-13.0661, -20.6138) ccw
  arc A301 (-14.0201, -20.6138) -> (-12.1121, -20.6138) centre (-13.0661, -20.6138) ccw
  arc A302 (-12.1121, -20.6138) -> (-14.0201, -20.6138) centre (-13.0661, -20.6138) ccw
  arc A303 (-14.3996, -20.6138) -> (-11.7326, -20.6138) centre (-13.0661, -20.6138) ccw
  arc A304 (-11.7326, -20.6138) -> (-14.3996, -20.6138) centre (-13.0661, -20.6138) ccw
  arc A305 (17.2234, -20.6138) -> (14.5564, -20.6138) centre (15.8899, -20.6138) ccw
  arc A306 (14.5564, -20.6138) -> (17.2234, -20.6138) centre (15.8899, -20.6138) ccw
  arc A307 (16.8439, -20.6138) -> (14.9359, -20.6138) centre (15.8899, -20.6138) ccw
  arc A308 (14.9359, -20.6138) -> (16.8439, -20.6138) centre (15.8899, -20.6138) ccw
  arc A309 (16.8439, -20.6138) -> (14.9359, -20.6138) centre (15.8899, -20.6138) ccw
  arc A310 (14.9359, -20.6138) -> (16.8439, -20.6138) centre (15.8899, -20.6138) ccw
  arc A311 (17.2234, -20.6138) -> (14.5564, -20.6138) centre (15.8899, -20.6138) ccw
  arc A312 (14.5564, -20.6138) -> (17.2234, -20.6138) centre (15.8899, -20.6138) ccw
  line L128 (-13.6281, -10.5648) -> (-12.6281, -10.5648)
  line L129 (-12.6281, -10.5648) -> (-12.6281, -11.5648)
  line L130 (-12.6281, -11.5648) -> (-13.6281, -11.5648)
  line L131 (-13.6281, -11.5648) -> (-13.6281, -10.5648)
  line L132 (-13.6281, -7.5648) -> (-12.6281, -7.5648)
  line L133 (-12.6281, -7.5648) -> (-12.6281, -8.5648)
  line L134 (-12.6281, -8.5648) -> (-13.6281, -8.5648)
  line L135 (-13.6281, -8.5648) -> (-13.6281, -7.5648)
  line L136 (-15.0281, -7.5648) -> (-14.0281, -7.5648)
  line L137 (-14.0281, -7.5648) -> (-14.0281, -8.5648)
  line L138 (-14.0281, -8.5648) -> (-15.0281, -8.5648)
  line L139 (-15.0281, -8.5648) -> (-15.0281, -7.5648)
  line L140 (-15.0281, -10.5648) -> (-14.0281, -10.5648)
  line L141 (-14.0281, -10.5648) -> (-14.0281, -11.5648)
  line L142 (-14.0281, -11.5648) -> (-15.0281, -11.5648)
  line L143 (-15.0281, -11.5648) -> (-15.0281, -10.5648)
  line L144 (18.4904, -14.0214) -> (17.7833, -14.7285)
  line L145 (17.7833, -14.7285) -> (17.0762, -14.0214)
  line L146 (17.0762, -14.0214) -> (17.7833, -13.3143)
  line L147 (17.7833, -13.3143) -> (18.4904, -14.0214)
  line L148 (16.2276, -16.2842) -> (15.5205, -16.9913)
  line L149 (15.5205, -16.9913) -> (14.8134, -16.2842)
  line L150 (14.8134, -16.2842) -> (15.5205, -15.5771)
  line L151 (15.5205, -15.5771) -> (16.2276, -16.2842)
  line L152 (-12.6967, -16.9913) -> (-13.4038, -16.2842)
  line L153 (-13.4038, -16.2842) -> (-12.6967, -15.5771)
  line L154 (-12.6967, -15.5771) -> (-11.9896, -16.2842)
  line L155 (-11.9896, -16.2842) -> (-12.6967, -16.9913)
  line L156 (-14.9595, -14.7285) -> (-15.6666, -14.0214)
  line L157 (-15.6666, -14.0214) -> (-14.9595, -13.3143)
  line L158 (-14.9595, -13.3143) -> (-14.2524, -14.0214)
  line L159 (-14.2524, -14.0214) -> (-14.9595, -14.7285)
  arc A313 (-8.5881, -16.645) -> (-8.5881, -14.4225) centre (-8.5881, -15.5338) ccw
  arc A314 (-8.5881, -14.4225) -> (-8.5881, -16.645) centre (-8.5881, -15.5338) ccw
  arc A315 (-8.5881, -16.4228) -> (-8.5881, -14.6448) centre (-8.5881, -15.5338) ccw
  arc A316 (-8.5881, -14.6448) -> (-8.5881, -16.4228) centre (-8.5881, -15.5338) ccw
  arc A317 (-8.5881, -16.4228) -> (-8.5881, -14.6448) centre (-8.5881, -15.5338) ccw
  arc A318 (-8.5881, -14.6448) -> (-8.5881, -16.4228) centre (-8.5881, -15.5338) ccw
  arc A319 (-8.5881, -16.645) -> (-8.5881, -14.4225) centre (-8.5881, -15.5338) ccw
  arc A320 (-8.5881, -14.4225) -> (-8.5881, -16.645) centre (-8.5881, -15.5338) ccw
  arc A321 (11.4119, -16.645) -> (11.4119, -14.4225) centre (11.4119, -15.5338) ccw
  arc A322 (11.4119, -14.4225) -> (11.4119, -16.645) centre (11.4119, -15.5338) ccw
  arc A323 (11.4119, -16.4228) -> (11.4119, -14.6448) centre (11.4119, -15.5338) ccw
  arc A324 (11.4119, -14.6448) -> (11.4119, -16.4228) centre (11.4119, -15.5338) ccw
  arc A325 (11.4119, -16.4228) -> (11.4119, -14.6448) centre (11.4119, -15.5338) ccw
  arc A326 (11.4119, -14.6448) -> (11.4119, -16.4228) centre (11.4119, -15.5338) ccw
  arc A327 (11.4119, -16.645) -> (11.4119, -14.4225) centre (11.4119, -15.5338) ccw
  arc A328 (11.4119, -14.4225) -> (11.4119, -16.645) centre (11.4119, -15.5338) ccw
  point P0 (2.8237, 0)
  constraints: 658 point on circle, 329 centre point, 320 end point, 4 symmetric about line, 4 other
sketch "スケッチ18" plane through (0, 0, 0) normal (0, 0, -1) x (-1, 0, 0)
  line L0 (-21.4196, 41.881) -> (24.2804, 41.881)
  line L1 (24.2804, 41.881) -> (24.2804, 20.581)
  line L2 (24.2804, 20.581) -> (-21.4196, 20.581)
  line L3 (-21.4196, 20.581) -> (-21.4196, 41.881)
  circle A0 centre (-18.9196, 39.381) radius 1.55
  circle A1 centre (21.7804, 23.081) radius 1.55
  circle A2 centre (-10.7696, 31.231) radius 8.15
  circle A3 centre (13.6304, 31.231) radius 8.15
  line L4 (19.1919, 20.5342) -> (-16.3681, 20.5342) projected
  point P0 (1.4304, 28.731)
  point P1 (1.4304, 28.731)
  constraints: 8 end point, 4 centre point
sketch "スケッチ21" plane through (0, 0, 0) normal (0, 0, -1) x (-1, 0, 0)
  line L0 (-21.4196, 20.581) -> (-21.4196, 41.881) projected
  arc A0 (-12.1121, -20.6138) -> (-14.0201, -20.6138) centre (-13.0661, -20.6138) ccw projected
  arc A1 (-14.0201, -20.6138) -> (-12.1121, -20.6138) centre (-13.0661, -20.6138) ccw projected
  arc A2 (14.9359, -20.6138) -> (16.8439, -20.6138) centre (15.8899, -20.6138) ccw projected
  arc A3 (16.8439, -20.6138) -> (14.9359, -20.6138) centre (15.8899, -20.6138) ccw projected
  circle A4 centre (-18.9196, 39.381) radius 1.55 projected
  circle A5 centre (21.7804, 23.081) radius 1.55 projected
  arc A6 (-8.2902, -23.9158) -> (-16.3681, -15.2115) centre (-21.4196, -28) ccw
  arc A7 (19.2289, -15.2115) -> (11.1509, -23.9158) centre (24.2804, -28) ccw
  line L1 (4.7797, 20.581) -> (4.7797, 15.1081)
  line L2 (5.7797, 14.1081) -> (13.9359, 14.1081)
  line L3 (14.9359, 13.1081) -> (14.9359, -0.6888)
  line L4 (-12.1121, 20.581) -> (-12.1121, -0.6888)
  line L5 (-16.3681, -15.2115) -> (-16.3681, -7.8183)
  line L6 (-16.3681, -0.6888) -> (-16.3681, 20.581)
  line L7 (-16.3681, -0.6888) -> (-12.1121, -0.6888)
  line L8 (14.9359, -0.6888) -> (19.2289, -0.6888)
  line L9 (19.2289, -15.2115) -> (19.2289, -7.8183)
  line L10 (19.2289, -0.6888) -> (19.2289, 20.581)
  line L11 (-14.3681, -5.8183) -> (-8.6023, -5.8183)
  line L12 (11.461, -5.8183) -> (17.2289, -5.8183)
  line L13 (-16.3681, 20.581) -> (-12.1121, 20.581)
  line L14 (4.7797, 20.581) -> (4.7797, 22.581)
  line L15 (4.7797, 22.581) -> (17.2289, 22.581)
  line L16 (19.2289, 20.581) -> (19.2289, 20.581)
  arc A8 (-8.6023, -5.8183) -> (-6.6023, -3.8183) centre (-8.6023, -3.8183) ccw
  arc A9 (9.461, -3.8183) -> (11.461, -5.8183) centre (11.461, -3.8183) ccw
  arc A10 (-14.3681, -5.8183) -> (-16.3681, -7.8183) centre (-14.3681, -7.8183) ccw
  arc A11 (19.2289, -7.8183) -> (17.2289, -5.8183) centre (17.2289, -7.8183) ccw
  arc A12 (19.2289, 20.581) -> (17.2289, 22.581) centre (17.2289, 20.581) ccw
  line L17 (-21.4196, 41.881) -> (-21.4196, -23.9158)
  line L18 (-21.4196, -23.9158) -> (-8.2902, -23.9158)
  line L19 (11.1509, -23.9158) -> (24.2804, -23.9158)
  line L20 (24.2804, 41.881) -> (-21.4196, 41.881)
  line L21 (9.461, -3.8183) -> (9.461, 11.1956)
  line L22 (8.461, 12.1956) -> (-5.6023, 12.1956)
  line L23 (-6.6023, 11.1956) -> (-6.6023, -3.8183)
  line L24 (24.2804, -23.9158) -> (24.2804, 41.881)
  line L25 (-50.2429, 1.6271) -> (8.6618, 1.6271) construction
  line L26 (-2.214, 29.5622) -> (-10.3349, 24.8736)
  line L27 (-14.3129, 27.1703) -> (-14.3129, 36.5475)
  line L28 (-10.3349, 38.8442) -> (-2.214, 34.1556)
  arc A13 (-14.3129, 27.1703) -> (-10.3349, 24.8736) centre (-11.6609, 27.1703) ccw
  arc A14 (-10.3349, 38.8442) -> (-14.3129, 36.5475) centre (-11.6609, 36.5475) ccw
  arc A15 (-2.214, 29.5622) -> (-2.214, 34.1556) centre (-3.54, 31.8589) ccw
  line L29 (5.0747, 29.5622) -> (13.1956, 24.8736)
  line L30 (17.1736, 27.1703) -> (17.1736, 36.5475)
  line L31 (13.1956, 38.8442) -> (5.0747, 34.1556)
  arc A16 (13.1956, 24.8736) -> (17.1736, 27.1703) centre (14.5216, 27.1703) ccw
  arc A17 (17.1736, 36.5475) -> (13.1956, 38.8442) centre (14.5216, 36.5475) ccw
  arc A18 (5.0747, 34.1556) -> (5.0747, 29.5622) centre (6.4007, 31.8589) ccw
  line L32 (0.9321, 34.4415) -> (-5.7024, 38.2515)
  line L33 (-5.2045, 40.1187) -> (1.4303, 40.1187)
  line L34 (1.9281, 34.4415) -> (8.5629, 38.251)
  line L35 (8.0651, 40.1182) -> (1.4303, 40.1187)
  arc A19 (-5.2045, 40.1187) -> (-5.7024, 38.2515) centre (-5.2045, 39.1187) ccw
  arc A20 (0.9321, 34.4415) -> (1.9281, 34.4415) centre (1.4301, 35.3087) ccw
  arc A21 (8.5629, 38.251) -> (8.0651, 40.1182) centre (8.065, 39.1182) ccw
  line L36 (0.9321, 29.2762) -> (-5.7024, 25.4663)
  line L37 (-5.2045, 23.5991) -> (1.4303, 23.5991)
  line L38 (8.0651, 23.5996) -> (1.4303, 23.5991)
  line L39 (1.9281, 29.2763) -> (8.5629, 25.4668)
  arc A22 (-5.7024, 25.4663) -> (-5.2045, 23.5991) centre (-5.2045, 24.5991) ccw
  arc A23 (1.9281, 29.2763) -> (0.9321, 29.2762) centre (1.4301, 28.409) ccw
  arc A24 (8.0651, 23.5996) -> (8.5629, 25.4668) centre (8.065, 24.5996) ccw
  arc A25 (14.9359, 13.1081) -> (13.9359, 14.1081) centre (13.9359, 13.1081) ccw
  arc A26 (4.7797, 15.1081) -> (5.7797, 14.1081) centre (5.7797, 15.1081) ccw
  arc A27 (9.461, 11.1956) -> (8.461, 12.1956) centre (8.461, 11.1956) ccw
  arc A28 (-5.6023, 12.1956) -> (-6.6023, 11.1956) centre (-5.6023, 11.1956) ccw
  line L40 (-21.4196, -23.9158) -> (24.2059, -23.9158)
  line L41 (24.2059, -23.9158) -> (24.2059, -26.6158)
  line L42 (24.2059, -26.6158) -> (-21.4196, -26.6158)
  line L43 (-21.4196, -26.6158) -> (-21.4196, -23.9158)
  point P0 (12.2118, 1.6271)
  point P1 (0.46, 31.8589)
  point P2 (-11.6644, 24.8589)
  point P3 (-14.3129, 41.1409)
  point P4 (2.4007, 31.8589)
  point P5 (14.5251, 24.8589)
  point P6 (17.1736, 41.1409)
  dimension "d65" = 27.5
  dimension "d66" = 27.5
  dimension "d68" = 2
  dimension "d73" = 2.652
  dimension "d74" = 1
  dimension "d75" = 1
  dimension "d76" = 2.7
  constraints: 86 end point, 46 point on circle, 28 tangent, 23 centre point, 13 perpendicular, 10 equal radius, 8 horizontal, 6 vertical, 4 parallel, 4 point on line
  measures "d65" diameter of A6
  measures "d66" diameter of A7
  measures "d68" radius of A8
  measures "d73" radius of A13
  measures "d74" radius of A19
  measures "d75" radius of A25
  measures "d76" distance of L40.end L41.end
extrude "押し出し12" add sketch "スケッチ21" against normal blind 3 contours L0 L20 L24 L19 A7 L9 A11 L12 A9 L21 A27 L22 A28 L23 A8 L11 A10 L5 A6 L18 L17
sketch "スケッチ22" plane through (0, 0, 0) normal (0, 0, -1) x (-1, 0, 0)
  line L0 (24.2059, -23.9158) -> (24.2059, -26.6158) projected
  line L1 (24.2059, -26.6158) -> (-21.4196, -26.6158) projected
  line L2 (-21.4196, -23.9158) -> (24.2059, -23.9158) projected
  line L3 (-21.4196, -26.6158) -> (-21.4196, -23.9158) projected
  point P0 (0, 0)
extrude "押し出し13" add sketch "スケッチ22" against normal blind 18
chamfer "面取り3" distance 1 angle 45 2 edges at (-17.6784, -23.9158, 3) (14.8549, -23.9158, 3)
sketch "スケッチ23" plane through (-11.1509, -23.9158, 0) normal (0, 1, 0) x (1, 0, 0)
  point P0 (11.1509, 0)
sketch "スケッチ24" plane through (-11.1509, -23.9158, 0) normal (0, 1, 0) x (1, 0, 0)
  circle A0 centre (-8.455, -14) radius 1.8
  line L0 (32.5706, -18) -> (-13.055, -18) projected
  line L1 (-13.055, -4) -> (-13.055, -18) projected
  circle A1 centre (-8.455, -8) radius 1.75
  line L2 (-13.055, 0) -> (32.5706, 0) projected
  circle A2 centre (28.0706, -14) radius 1.75
  line L3 (32.5706, -4) -> (32.5706, -18) projected
  circle A3 centre (28.0706, -8) radius 1.75
  point P0 (11.1509, 0)
  dimension "d84" = 3.6
  dimension "d85" = 4
  dimension "d86" = 4.6
  dimension "d87" = 3.5
  dimension "d88" = 8
  dimension "d89" = 3.5
  dimension "d90" = 4.5
  dimension "d91" = 3.5
  constraints: 4 centre point
  measures "d84" diameter of A0
  measures "d85" distance from line of L0 A0.centre
  measures "d86" distance from line of L1 A0.centre
  measures "d87" diameter of A1
  measures "d88" distance from line of L2 A1.centre
  measures "d89" diameter of A2
  measures "d90" distance from line of L3 A2.centre
  measures "d91" diameter of A3
extrude "押し出し14" cut sketch "スケッチ24" against normal blind 2.7
sketch "スケッチ25" plane through (-11.1509, -23.9158, 0) normal (0, 1, 0) x (1, 0, 0)
  line L0 (-13.055, -18) -> (32.5706, -18) projected
  line L1 (-13.055, 0) -> (32.5706, 0) projected
  line L2 (8.6573, 0) -> (8.6573, -18)
  line L3 (10.8583, 0) -> (10.8583, -18)
  line L4 (8.6573, 0) -> (10.8583, 0)
  line L5 (19.4412, 0) -> (0, 0) projected
  line L6 (8.6573, -18) -> (10.8583, -18)
  line L7 (32.5706, -18) -> (-13.055, -18) projected
  point P0 (11.1509, 0)
  constraints: 8 end point, 2 collinear, 1 point on line, 1 vertical
extrude "押し出し15" cut sketch "スケッチ25" against normal blind 1
chamfer "面取り4" distance 0.1 angle 45 2 edges at (-2.4936, -24.9158, 9) (-0.2927, -24.9158, 9)
